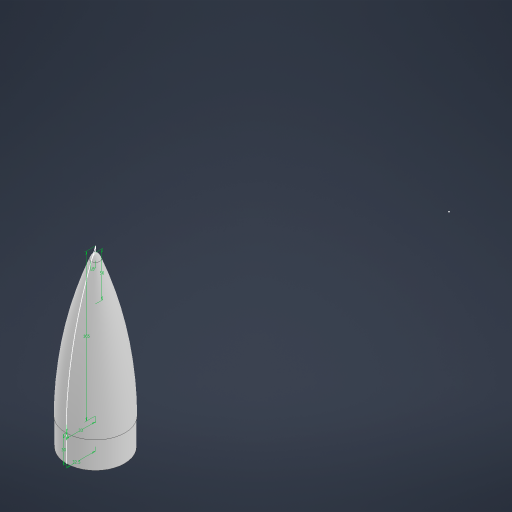
# Autodesk Inventor part: nosecone bt80
Saved by Autodesk Inventor 2024 (Build 280153000, 153)
## iProperties
Created: 2025-02-25
Part Number: nosecone bt80
Material: Generic
Document SubType Name: Modeling
Designer: huj31
Density: 1 g/cm^3
Appearance: Default
Author: huj31
Autodesk Inventor part; units mm, degrees
ref_plane "YZ Plane" through (0, 0, 0) normal (1, 0, 0) x (0, 1, 0)
ref_plane "XZ Plane" through (0, 0, 0) normal (0, 1, 0) x (-1, 0, 0)
ref_plane "XY Plane" through (0, 0, 0) normal (0, 0, 1) x (1, 0, 0)
sketch "Sketch1" plane through (0, 0, 0) normal (1, 0, 0) x (0, 1, 0)
  line L0 (0, 0) -> (-30, 0)
  line L1 (-30, 0) -> (-30, 32.5)
  line L2 (-30, 32.5) -> (0, 32.5)
  line L3 (0, 32.5) -> (0, 0)
  line L4 (0, 0) -> (0, 33)
  line L5 (0, 0) -> (165, 0)
  arc A0 (165, 0) -> (0, 33) centre (0, -396) ccw
  ellipse E0 centre (108.5922, 0) end of major axis (158.5922, 0) minor radius 10.4096 (158.5922, 0) -> (152.4467, 5) ccw
  line L6 (152.4467, 5) -> (150.5459, 0)
  point P0 (0, 32.5)
  dimension "d8" = 50
  dimension "d0" = 30
  dimension "d1" = 32.5
  dimension "d2" = 33
  dimension "d3" = 165
  dimension "d10" = 5
  dimension "d13" = 0
  constraints: 14 end point, 4 point on circle, 3 point on line, 2 horizontal, 2 line through centre, 2 parallel, 2 perpendicular, 1 centre point, 1 vertical, 6 other
  measures "d0" distance of L1.end L2.end
  measures "d1" distance of L0.end L1.end
  measures "d2" distance of L0.start L4.end
  measures "d3" distance of L0.start L5.end
  measures "d10" vertical distance of L6.start L6.end
  measures "d13" distance from line of point (0, 32.5) L4
revolve "Revolution1" add sketch "Sketch1" angle 360 about axis through (0, 0, 0) along (0, 1, 0) contours L0 L1 L2 L3 | L3 L4 A0 L6 L5 | L6 E0 L5
body "Solid1"
